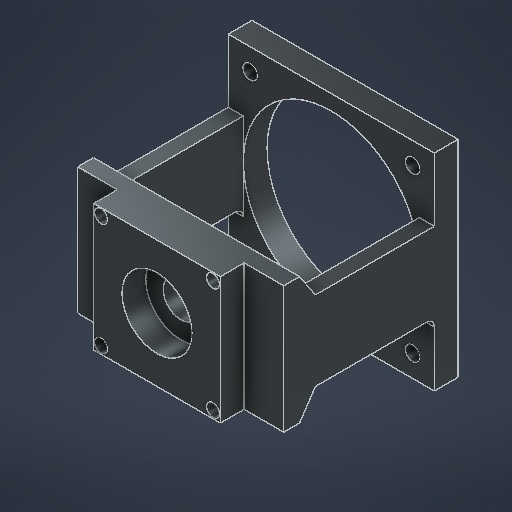
# Autodesk Inventor part: MOTOR-BRACKET
Saved by Autodesk Inventor 2025.3 (Build 293356030, 356C)
## iProperties
Created: 2025-09-29
Part Number: MOTOR-BRACKET
Material: Generic
Document SubType Name: Modeling
Designer: lstk1ng
Density: 1 g/cm^3
Appearance: Iron Gray
Author: lstk1ng
Autodesk Inventor part; units mm, degrees
note: some values were not read from the file. Chosen so that the rebuilt part matches the saved one: edges of "Fillet1".
ref_plane "YZ Plane" through (0, 0, 0) normal (1, 0, 0) x (0, 1, 0)
ref_plane "XZ Plane" through (0, 0, 0) normal (0, 1, 0) x (-1, 0, 0)
ref_plane "XY Plane" through (0, 0, 0) normal (0, 0, 1) x (1, 0, 0)
sketch "Sketch1" plane through (0, 0, 0) normal (0, 0, 1) x (1, 0, 0)
  line L0 (-65, 65) -> (65, 65)
  line L1 (65, 65) -> (65, -65)
  line L2 (65, -65) -> (-65, -65)
  line L3 (-65, -65) -> (-65, 65)
  line L4 (-65, 65) -> (65, -65) construction
  line L5 (65, 65) -> (-65, -65) construction
  circle A0 centre (0, 0) radius 72.5 construction
  circle A1 centre (51.2652, 51.2652) radius 4.5
  line L6 (0, 0) -> (0, 13.8436) construction
  line L7 (0, 0) -> (-14.1522, 0) construction
  circle A2 centre (-51.2652, 51.2652) radius 4.5
  circle A3 centre (51.2652, -51.2652) radius 4.5
  circle A4 centre (-51.2652, -51.2652) radius 4.5
  dimension "d66" = 145
  dimension "d0" = 130
  dimension "d1" = 130
  dimension "d67" = 9
  constraints: 16 end point, 4 centre point, 3 symmetric about line, 2 horizontal, 2 midpoint, 2 parallel, 1 coincident, 1 perpendicular, 1 point on line, 1 vertical, 6 other
  measures "d0" distance of L1.end L2.end
  measures "d1" distance of L0.end L1.end
  measures "d67" diameter of A1
extrude "Extrusion1" add sketch "Sketch1" along normal blind 15
sketch "Sketch2" plane through (65, -65, 0) normal (1, 0, 0) x (0, 0, -1)
  line L0 (0, 0) -> (0, 130) construction
  line L1 (-22.5, 65) -> (-82.5, 65) construction
  line L2 (-90, 40) -> (-15, 40)
  line L3 (-15, 90) -> (-15, 40)
  line L4 (-15, 0) -> (-15, 130) construction
  line L5 (-15, 90) -> (-15, 130) construction
  line L6 (-100, 105) -> (-110, 105)
  line L7 (-110, 105) -> (-110, 25)
  line L8 (-15, 90) -> (-90, 90)
  line L9 (-90, 90) -> (-100, 105)
  line L10 (-110, 25) -> (-100, 25)
  line L11 (-100, 25) -> (-90, 40)
  point P0 (0, 90)
  point P1 (0, 40)
  dimension "d98" = 10
  dimension "d101" = 110
  dimension "d102" = 75
  dimension "d103" = 75
  dimension "d104" = 10
  constraints: 20 end point, 3 horizontal, 2 perpendicular, 1 collinear, 1 point on line, 1 symmetric about line
  measures "d98" distance of L6.start L6.end
  measures "d101" distance between parallel lines of L0 L7
  measures "d102" distance of L5.start L8.end
  measures "d103" distance of L2.start L2.end
  measures "d104" distance of L7.end L10.end
extrude "Extrusion2" add sketch "Sketch2" against normal blind 9.5
mirror "Mirror1" about plane through (0, 0, 0) normal (1, 0, 0) of "Extrusion2"
sketch "Sketch6" plane through (0, 0, 0) normal (0, 0, -1) x (-1, 0, 0)
  circle A0 centre (0, 0) radius 55.5
  dimension "d37" = 111
  constraints: 1 centre point, 1 coincident
  measures "d37" diameter of A0
extrude "Extrusion6" cut sketch "Sketch6" against normal up to surface (15 mm away)
fillet "Fillet1" radius 5 2 edges at (-60.25, -25, 15) (60.25, -25, 15)
sketch "Sketch14" plane through (-65, -40, 110) normal (0, 0, 1) x (1, 0, 0)
  line L0 (120.5, 15) -> (120.5, 0) projected
  line L1 (9.5, 80) -> (120.5, 80)
  line L2 (120.5, 80) -> (120.5, 0)
  line L3 (120.5, 0) -> (9.5, 0)
  line L4 (9.5, 0) -> (9.5, 80)
  constraints: 8 end point, 2 parallel, 1 horizontal, 1 perpendicular
extrude "Extrusion14" add sketch "Sketch14" against normal blind 10
sketch "Sketch15" plane through (65, -40, 110) normal (0, 0, 1) x (1, 0, 0)
  line L0 (-25, 0) -> (-105, 0)
  line L1 (-105, 0) -> (-105, 80)
  line L2 (-105, 80) -> (-25, 80)
  line L3 (-25, 80) -> (-25, 0)
  line L4 (-25, 0) -> (-105, 80) construction
  line L5 (-105, 0) -> (-25, 80) construction
  point P0 (-65, 40)
  dimension "d105" = 80
  dimension "d106" = 80
  constraints: 12 end point, 2 midpoint, 2 parallel, 1 horizontal, 1 perpendicular
  measures "d105" distance of L1.end L2.end
  measures "d106" distance of L0.end L1.end
extrude "Extrusion15" add sketch "Sketch15" along normal blind 15
sketch "Sketch16" plane through (65, -40, 125) normal (0, 0, 1) x (1, 0, 0)
  circle A0 centre (-65, 40) radius 50 construction
  line L0 (-65, 40) -> (-100.3553, 75.3553) construction
  line L1 (-65, 40) -> (-15, 40) construction
  line L2 (-65, 40) -> (-65, 52) construction
  circle A1 centre (-100.3553, 75.3553) radius 4.075
  circle A2 centre (-29.6447, 75.3553) radius 4.075
  circle A3 centre (-100.3553, 4.6447) radius 4.075
  circle A4 centre (-29.6447, 4.6447) radius 4.075
  circle A5 centre (-65, 40) radius 11.075
  dimension "d109" = 100
  dimension "d110" = 135
  dimension "d111" = 12
  dimension "d112" = 8.15
  dimension "d113" = 22.15
  constraints: 6 end point, 5 centre point, 3 coincident, 3 symmetric about line, 1 equal length, 1 horizontal, 1 vertical, 6 other
  measures "d110" angle of L1 L0
  measures "d111" distance of L0.start L2.end
  measures "d112" diameter of A1
  measures "d113" diameter of A5
extrude "Extrusion16" cut sketch "Sketch16" against normal up to surface (25 mm away)
sketch "Sketch17" plane through (65, -40, 125) normal (0, 0, 1) x (1, 0, 0)
  circle A0 centre (-65, 40) radius 22.05
  circle A1 centre (-65, 40) radius 11.075 projected
  dimension "d116" = 44.1
  constraints: 1 centre point, 1 coincident
  measures "d116" diameter of A0
extrude "Extrusion17" cut sketch "Sketch17" against normal blind 15
body "Solid1"
